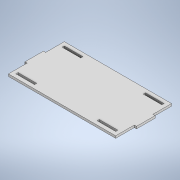
# Autodesk Inventor part: Level1 (Motoren)
Saved by Autodesk Inventor 2020 (Build 240168000, 168)
## iProperties
Created: 2020-01-30
Part Number: Level1 (Motoren)
Material: Generic
Document SubType Name: Modeling
Designer: jelte
Density: 1 g/cm^3
Appearance: Default
Mass: 31.5475 g
Surface Area: 230.707 cm^2
Volume: 31.5475 cm^3
Author: jelte
Autodesk Inventor part; units mm, degrees
ref_plane "YZ Plane" through (0, 0, 0) normal (1, 0, 0) x (0, 1, 0)
ref_plane "XZ Plane" through (0, 0, 0) normal (0, 1, 0) x (-1, 0, 0)
ref_plane "XY Plane" through (0, 0, 0) normal (0, 0, 1) x (1, 0, 0)
sketch "Sketch1" plane through (0, 0, 0) normal (0, 1, 0) x (-1, 0, 0)
  line L0 (71.1097, -38.0648) -> (71.1097, -13.0648)
  line L1 (71.1097, -13.0648) -> (74.1097, -13.0648)
  line L2 (74.1097, -13.0648) -> (74.1097, 11.9352)
  line L3 (74.1097, 11.9352) -> (71.1097, 11.9352)
  line L4 (71.1097, 11.9352) -> (71.1097, 36.9352)
  line L5 (-72.8903, -38.0648) -> (-72.8903, -13.0648)
  line L6 (-72.8903, 36.9352) -> (-72.8903, 11.9352)
  line L7 (-72.8903, -13.0648) -> (-75.8903, -13.0648)
  line L8 (-75.8903, -13.0648) -> (-75.8903, 11.9352)
  line L9 (-75.8903, 11.9352) -> (-72.8903, 11.9352)
  line L10 (71.1097, -38.0648) -> (-72.8903, -38.0648)
  line L11 (71.1097, 36.9352) -> (-72.8903, 36.9352)
  point P0 (0, 0)
  constraints: 24 end point, 5 perpendicular, 3 horizontal, 2 vertical
extrude "Extrusion1" add sketch "Sketch1" along normal blind 3
sketch "Sketch2" plane through (0, 3, 0) normal (0, 1, 0) x (1, 0, 0)
  line L0 (-71.1097, -36.9352) -> (72.8903, -36.9352) projected
  line L1 (-66.1097, -31.9352) -> (-56.1097, -31.9352)
  line L2 (-56.1097, -31.9352) -> (-56.1097, -28.9352)
  line L3 (-56.1097, -28.9352) -> (-66.1097, -28.9352)
  line L4 (-66.1097, -28.9352) -> (-66.1097, -31.9352)
  line L5 (72.8903, 38.0648) -> (-71.1097, 38.0648) projected
  line L6 (-56.1097, 30.0648) -> (-66.1097, 30.0648)
  line L7 (-66.1097, 30.0648) -> (-66.1097, 33.0648)
  line L8 (-66.1097, 33.0648) -> (-56.1097, 33.0648)
  line L9 (-56.1097, 33.0648) -> (-56.1097, 30.0648)
  line L10 (67.8903, 33.0648) -> (57.8903, 33.0648)
  line L11 (57.8903, 33.0648) -> (57.8903, 30.0648)
  line L12 (57.8903, 30.0648) -> (67.8903, 30.0648)
  line L13 (67.8903, 30.0648) -> (67.8903, 33.0648)
  line L14 (67.8903, -31.9352) -> (57.8903, -31.9352)
  line L15 (57.8903, -31.9352) -> (57.8903, -28.9352)
  line L16 (57.8903, -28.9352) -> (67.8903, -28.9352)
  line L17 (67.8903, -28.9352) -> (67.8903, -31.9352)
  point P0 (0, 0)
  constraints: 32 end point, 8 parallel, 4 horizontal, 4 perpendicular, 1 point on line
extrude "Extrusion2" cut sketch "Sketch2" against normal blind 30
sketch "Sketch3" plane through (0, 3, 0) normal (0, 1, 0) x (1, 0, 0)
  line L0 (72.8903, 38.0648) -> (-71.1097, 38.0648) projected
  circle A0 centre (-14.1097, 28.0648) radius 5
  circle A1 centre (15.8903, 28.0648) radius 5
  line L1 (-71.1097, -36.9352) -> (72.8903, -36.9352) projected
  circle A2 centre (-14.1097, -26.9352) radius 5
  circle A3 centre (15.8903, -26.9352) radius 5
  point P0 (0, 0)
  dimension "d35" = 10
  dimension "d36" = 10
  dimension "d39" = 10
  dimension "d40" = 10
  constraints: 4 centre point
  measures "d35" diameter of A0
  measures "d36" diameter of A1
  measures "d39" diameter of A2
  measures "d40" diameter of A3
extrude "Extrusion3" cut sketch "Sketch3" against normal blind 30
sketch "Sketch4" plane through (0, 3, 0) normal (0, 1, 0) x (1, 0, 0)
  line L0 (-56.1097, 33.0648) -> (-56.1097, 30.0648) projected
  line L1 (-56.1097, 33.0648) -> (-41.1097, 33.0648)
  line L2 (-41.1097, 33.0648) -> (-41.1097, 30.0648)
  line L3 (-41.1097, 30.0648) -> (-56.1097, 30.0648)
  line L4 (-56.1097, 30.0648) -> (-56.1097, 33.0648)
  line L5 (57.8903, 33.0648) -> (42.8903, 33.0648)
  line L6 (42.8903, 33.0648) -> (42.8903, 30.0648)
  line L7 (42.8903, 30.0648) -> (57.8903, 30.0648)
  line L8 (57.8903, 30.0648) -> (57.8903, 33.0648)
  line L9 (-56.1097, -31.9352) -> (-66.1097, -31.9352) projected
  line L10 (-56.1097, -31.9352) -> (-41.1097, -31.9352)
  line L11 (-41.1097, -31.9352) -> (-41.1097, -28.9352)
  line L12 (-41.1097, -28.9352) -> (-56.1097, -28.9352)
  line L13 (-56.1097, -28.9352) -> (-56.1097, -31.9352)
  line L14 (57.8903, -31.9352) -> (57.8903, -28.9352) projected
  line L15 (57.8903, -31.9352) -> (42.8903, -31.9352)
  line L16 (42.8903, -31.9352) -> (42.8903, -28.9352)
  line L17 (42.8903, -28.9352) -> (57.8903, -28.9352)
  line L18 (57.8903, -28.9352) -> (57.8903, -31.9352)
  point P0 (0, 0)
  dimension "d43" = 15
  dimension "d44" = 15
  constraints: 32 end point, 8 parallel, 4 horizontal, 4 perpendicular, 1 point on line
  measures "d43" distance of L2.end L3.end
  measures "d44" distance of L5.start L5.end
extrude "Extrusion4" cut sketch "Sketch4" against normal blind 10
sketch "Sketch5" plane through (0, 3, 0) normal (0, 1, 0) x (1, 0, 0)
  circle A0 centre (-14.1097, 28.0648) radius 5 projected
  circle A1 centre (-14.1097, 28.0648) radius 5
  circle A2 centre (15.8903, 28.0648) radius 5 projected
  circle A3 centre (15.8903, 28.0648) radius 5
  circle A4 centre (15.8903, -26.9352) radius 5 projected
  circle A5 centre (15.8903, -26.9352) radius 5
  circle A6 centre (-14.1097, -26.9352) radius 5 projected
  circle A7 centre (-14.1097, -26.9352) radius 5
  point P0 (0, 0)
  constraints: 4 centre point, 4 coincident
extrude "Extrusion5" add sketch "Sketch5" against normal blind 3
body "Solid1"
